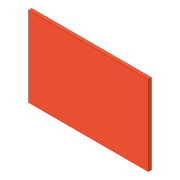
# Autodesk Inventor part: Generic8inFloor0
Saved by Autodesk Inventor 2019.4 (Build 234330000, 330)
## iProperties
Created: 2020-07-27
Part Number: Generic8inFloor0
Material: -=Choose Material=-
Document SubType Name: Modeling
Designer: sanchezb-1
Mass: 0.48 g
Surface Area: 1280 cm^2
Volume: 480 cm^3
Density: 0.001 g/cm^3
Appearance: Choose Color
Author: sanchezb-1
Mass (kg): 0.001
Spare Part: False
is ECP and relevant for alignment: False
is EDA Placeholder: False
Make AND Buy: False
Commercial off the Shelf: False
Autodesk Inventor part; units mm, degrees
ref_plane "YZ Plane" through (0, 0, 0) normal (1, 0, 0) x (0, 1, 0)
ref_plane "XZ Plane" through (0, 0, 0) normal (0, 1, 0) x (-1, 0, 0)
ref_plane "XY Plane" through (0, 0, 0) normal (0, 0, 1) x (1, 0, 0)
sketch "Sketch1" plane through (0, 0, 0) normal (0, 1, 0) x (-1, 0, 0)
  line L0 (0, 0) -> (0, 200)
  line L1 (0, 200) -> (300, 200)
  line L2 (300, 200) -> (300, 0)
  line L3 (300, 0) -> (0, 0)
  dimension "d0" = 200
  dimension "d1" = 300
  constraints: 8 end point
  measures "d0" distance of L0.start L0.end
  measures "d1" distance of L0.end L1.end
extrude "Extrusion1" add sketch "Sketch1" along normal blind 8
equation "\"PointX0\" = 0"
equation "\"PointY0\" = 0"
equation "\"PointZ0\" = 0"
equation "\"PointX1\" = 0"
equation "\"PointZ1\" = 0"
equation "\"PointZ2\" = 0"
equation "\"PointY3\" = 0"
equation "\"PointZ3\" = 0"
equation "\"length\" = 8"
body "Solid1"
